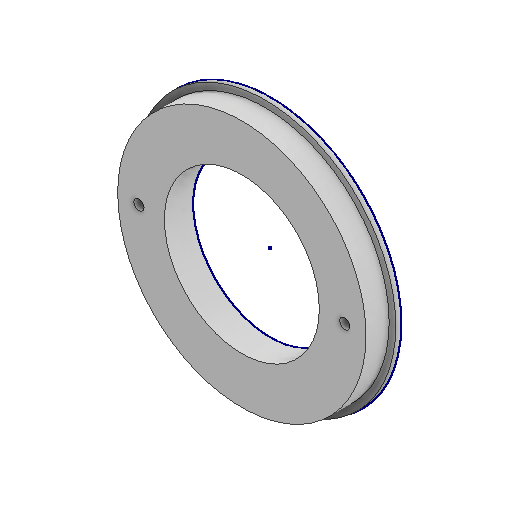
# Autodesk Inventor part: Adapter-MitutoyoMT1-SM2
Saved by Autodesk Inventor 2023 (Build 270158000, 158)
## iProperties
Created: 2022-09-26
Part Number: Adapter-MitutoyoMT1-SM2
Material: Generic
Document SubType Name: Modeling
Designer: nvladi
Density: 1 g/cm^3
Appearance: Default
Author: nvladi
Autodesk Inventor part; units mm, degrees
ref_plane "YZ Plane" through (0, 0, 0) normal (1, 0, 0) x (0, 1, 0)
ref_plane "XZ Plane" through (0, 0, 0) normal (0, 1, 0) x (-1, 0, 0)
ref_plane "XY Plane" through (0, 0, 0) normal (0, 0, 1) x (1, 0, 0)
sketch "Sketch1" plane through (0, 0, 0) normal (0, 0, 1) x (1, 0, 0)
  circle A0 centre (0, 0) radius 15.05
  circle A1 centre (0, 0) radius 24.125
  circle A2 centre (0, 0) radius 25.4
  point P0 (-20, 0)
  point P1 (20, 0)
  dimension "d0" = 30.1
  dimension "d1" = 48.25
  dimension "d2" = 50.8
  constraints: 3 centre point, 3 coincident
  measures "d0" diameter of A0
  measures "d1" diameter of A1
  measures "d2" diameter of A2
extrude "Extrusion1" add sketch "Sketch1" along normal blind 5.5 contours A1
extrude "Extrusion2" add sketch "Sketch1" along normal blind 1 contours A2
hole "Hole1" at (-20, 0, 0) at (20, 0, 0) direction (0, 0, 1) diameter 2 end through all
body "Solid1"
